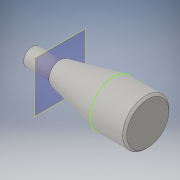
# Autodesk Inventor part: Kevin_CAD_test_2
Saved by Autodesk Inventor 2016 (Build 200138000, 138)
## iProperties
Created: 2018-06-19
Part Number: Kevin_CAD_test_2
Material: Generic
Document SubType Name: Modeling
Designer: Student
Density: 1 g/cm^3
Appearance: Default
Author: Student
Autodesk Inventor part; units mm, degrees
ref_plane "YZ Plane" through (0, 0, 0) normal (1, 0, 0) x (0, 1, 0)
ref_plane "XZ Plane" through (0, 0, 0) normal (0, 1, 0) x (-1, 0, 0)
ref_plane "XY Plane" through (0, 0, 0) normal (0, 0, 1) x (1, 0, 0)
sketch "Sketch1" plane through (0, 0, 0) normal (1, 0, 0) x (0, 1, 0)
  circle A0 centre (0, 0) radius 12.7
  dimension "d0" = 25.4
  constraints: 1 centre point, 1 coincident
  measures "d0" diameter of A0
extrude "Extrusion1" add sketch "Sketch1" along normal blind 19.05
chamfer "Chamfer1" distance 1.143 angle 45 1 edges at (19.05, -12.7, 0)
sketch "Sketch2" plane through (0, 0, 0) normal (-1, 0, 0) x (0, 0, 1)
  circle A0 centre (0, 0) radius 12.7
  constraints: 1 centre point, 1 coincident
ref_plane "Work Plane1" through (-29.21, 0, 0) normal (-1, 0, 0) x (0, 0, 1)
sketch "Sketch3" plane through (-29.21, 0, 0) normal (-1, 0, 0) x (0, 0, 1)
  circle A0 centre (0, 0) radius 6.096
  dimension "d7" = 12.192
  constraints: 1 centre point, 1 coincident
  measures "d7" diameter of A0
loft "Loft1" add profiles "Sketch3" section 1 edges at (0, -12.7, 0)
sketch "Sketch4" plane through (-29.21, 0, 0) normal (-1, 0, 0) x (0, 0, 1)
  circle A0 centre (0, 0) radius 4.7625
  dimension "d12" = 9.525
  constraints: 1 centre point, 1 coincident
  measures "d12" diameter of A0
extrude "Extrusion2" add sketch "Sketch4" along normal blind 15.24
body "Solid1"
